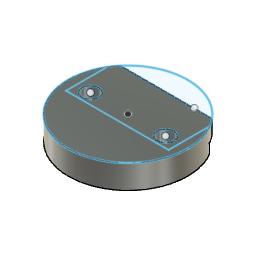
IMU - Platform v1 (Autodesk Fusion 360 design; units mm, degrees)
Autodesk Fusion 360 part; units mm, degrees
sketch "Sketch1" plane through (0, 0, 0) normal (0, 0, 1) x (1, 0, 0)
  circle A0 centre (0, 0) radius 12.5
  line L0 (-10, -2.2463) -> (-10.75, -2.2463)
  line L1 (-10.75, -2.2463) -> (-10.75, 6.3787)
  line L2 (10.75, -2.2463) -> (10.75, 6.3787)
  line L3 (5.8702, 8) -> (9.6047, 8) construction
  line L4 (10, -2.2463) -> (-10, -2.2463)
  circle A1 centre (-7.875, 0) radius 1.75
  line L5 (10, -2.2463) -> (10.75, -2.2463)
  line L6 (9.6047, 8) -> (-9.6047, 8)
  circle A2 centre (0, 0) radius 12.5
  circle A3 centre (7.875, 0) radius 1.75
  dimension "d1" = 25
  dimension "d10" = 3.5
  dimension "d11" = 3.5
  dimension "d20" = 0.75
  dimension "d21" = 0.75
  constraint coincident A0.centre A2.centre
  constraint coincident L1.end A2
  constraint perpendicular L0 L1
  constraint coincident L2.end A2
  constraint perpendicular L2 L5
  constraint coincident L3.end A2
  constraint coincident L6.end A2
  measures "d1" diameter of A0
  measures "d10" diameter of A3
  measures "d11" diameter of A1
  measures "d20" distance of L2.start L4.start
  measures "d21" distance of L0.end L0.start
extrude "Extrude1" add sketch "Sketch1" against normal blind 3 contours A0 L0 L1 L2 L4 L5 A2 | A0 L0 L1 L2 L4 L5 L6 A2
extrude "Extrude2" cut 1 faces at (-0.1963, -4.8192, -3) along direction (0, 0, 1) blind 3
extrude "Extrude3" add sketch "Sketch1" against normal blind 5 contours A0 L0 L1 L2 L4 L5 A2
extrude "Extrude4" add sketch "Sketch1" against normal blind 3 contours A0 L0 L1 L2 L4 L5 L6 A2
